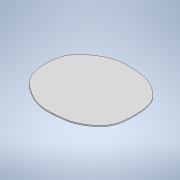
# Autodesk Inventor part: head_1
Saved by Autodesk Inventor 2020 (Build 240168000, 168)
## iProperties
Created: 2022-02-10
Part Number: head_1
Material: Типовые
Document SubType Name: Modeling
Designer: HP
Density: 1 g/cm^3
Appearance: По умолчанию
Author: HP
Autodesk Inventor part; units mm, degrees
ref_plane "YZ Plane" through (0, 0, 0) normal (1, 0, 0) x (0, 1, 0)
ref_plane "XZ Plane" through (0, 0, 0) normal (0, 1, 0) x (-1, 0, 0)
ref_plane "XY Plane" through (0, 0, 0) normal (0, 0, 1) x (1, 0, 0)
sketch "Эскиз1" plane through (0, 0, 0) normal (0, 1, 0) x (-1, 0, 0)
  line L0 (-81.3316, -22.101) -> (-82.4097, -10.5497) construction
  line L1 (-82.4097, -10.5497) -> (-83.3338, 3.774) construction
  line L2 (-83.3338, 3.774) -> (-82.2557, 21.486) construction
  line L3 (-82.2557, 21.486) -> (-81.3316, 38.8901) construction
  line L4 (-81.3316, 38.8901) -> (-79.8522, 51.3377) construction
  line L5 (-79.8522, 51.3377) -> (-76.1961, 64.7434) construction
  line L6 (-76.1961, 64.7434) -> (-73.0275, 74.6555) construction
  line L7 (-73.0275, 74.6555) -> (-68.2339, 84.2426) construction
  line L8 (-68.2339, 84.2426) -> (-63.1966, 91.2298) construction
  line L9 (-63.1966, 91.2298) -> (-56.2094, 98.7045) construction
  line L10 (-56.2094, 98.7045) -> (-49.8722, 104.8792) construction
  line L11 (-49.8722, 104.8792) -> (-42.6413, 111.5415) construction
  line L12 (-42.6413, 111.5415) -> (-35.4916, 118.0412) construction
  spline S0 degree 4 poles (-81.3316, -22.101) (-82.4097, -10.5497) (-83.3338, 3.774) (-82.2557, 21.486) (-81.3316, 38.8901) (-79.8522, 51.3377) (-76.1961, 64.7434) (-73.0275, 74.6555) (-68.2339, 84.2426) (-63.1966, 91.2298) (-56.2094, 98.7045) (-49.8722, 104.8792) (-42.6413, 111.5415) (-35.4916, 118.0412) knots 1 1 1 1 1 2 3 4 5 6 7 8 9 10 11 11 11 11 11
  line L13 (-35.4916, 118.0412) -> (-26.9213, 124.335) construction
  line L14 (-26.9213, 124.335) -> (-18.4284, 129.3436) construction
  line L15 (-18.4284, 129.3436) -> (-8.1934, 134.4974) construction
  line L16 (-8.1934, 134.4974) -> (-0.1361, 138.4897) construction
  line L17 (-0.1361, 138.4897) -> (9.5182, 142.1192) construction
  line L18 (9.5182, 142.1192) -> (19.245, 145.0227) construction
  line L19 (19.245, 145.0227) -> (26.7942, 146.4745) construction
  line L20 (26.7942, 146.4745) -> (34.6338, 147.7085) construction
  line L21 (34.6338, 147.7085) -> (42.183, 148.6521) construction
  line L22 (42.183, 148.6521) -> (49.8774, 149.6684) construction
  line L23 (49.8774, 149.6684) -> (59.0962, 150.9024) construction
  line L24 (59.0962, 150.9024) -> (68.823, 151.6283) construction
  line L25 (68.823, 151.6283) -> (77.4611, 152.2815) construction
  line L26 (77.4611, 152.2815) -> (85.0103, 152.2815) construction
  line L27 (85.0103, 152.2815) -> (93.1402, 152.9348) construction
  line L28 (93.1402, 152.9348) -> (101.4153, 152.9348) construction
  line L29 (101.4153, 152.9348) -> (111.5051, 151.5557) construction
  spline S1 degree 4 poles (-35.4916, 118.0412) (-26.9213, 124.335) (-18.4284, 129.3436) (-8.1934, 134.4974) (-0.1361, 138.4897) (9.5182, 142.1192) (19.245, 145.0227) (26.7942, 146.4745) (34.6338, 147.7085) (42.183, 148.6521) (49.8774, 149.6684) (59.0962, 150.9024) (68.823, 151.6283) (77.4611, 152.2815) (85.0103, 152.2815) (93.1402, 152.9348) (101.4153, 152.9348) (111.5051, 151.5557) knots 1 1 1 1 1 2 3 4 5 6 7 8 9 10 11 12 13 14 15 15 15 15 15
  line L30 (111.5051, 151.5557) -> (120.4722, 150.4408) construction
  line L31 (120.4722, 150.4408) -> (127.0223, 148.8843) construction
  line L32 (127.0223, 148.8843) -> (136.88, 145.7713) construction
  line L33 (136.88, 145.7713) -> (146.6728, 142.5287) construction
  line L34 (146.6728, 142.5287) -> (156.9196, 138.2484) construction
  line L35 (156.9196, 138.2484) -> (167.6204, 132.6061) construction
  line L36 (167.6204, 132.6061) -> (176.8944, 127.1585) construction
  line L37 (176.8944, 127.1585) -> (185.5199, 121.4514) construction
  line L38 (185.5199, 121.4514) -> (194.1438, 115.6177) construction
  spline S2 degree 4 poles (111.5051, 151.5557) (120.4722, 150.4408) (127.0223, 148.8843) (136.88, 145.7713) (146.6728, 142.5287) (156.9196, 138.2484) (167.6204, 132.6061) (176.8944, 127.1585) (185.5199, 121.4514) (194.1438, 115.6177) knots 1 1 1 1 1 2 3 4 5 6 7 7 7 7 7
  line L39 (194.1438, 115.6177) -> (200.24, 111.078) construction
  line L40 (200.24, 111.078) -> (206.9199, 106.0194) construction
  line L41 (206.9199, 106.0194) -> (214.1834, 99.9232) construction
  line L42 (214.1834, 99.9232) -> (219.8905, 93.2434) construction
  line L43 (219.8905, 93.2434) -> (226.1164, 84.3585) construction
  line L44 (226.1164, 84.3585) -> (232.2126, 74.7602) construction
  line L45 (232.2126, 74.7602) -> (234.0285, 71.4527) construction
  line L46 (234.0285, 71.4527) -> (236.5578, 65.162) construction
  line L47 (236.5578, 65.162) -> (240.1895, 53.5532) construction
  line L48 (240.1895, 53.5532) -> (243.1079, 38.7667) construction
  line L49 (243.1079, 38.7667) -> (244.9887, 26.8338) construction
  line L50 (244.9887, 26.8338) -> (246.2209, 14.4468) construction
  line L51 (246.2209, 14.4468) -> (246.2209, 2.9029) construction
  line L52 (246.2209, 2.9029) -> (245.2481, -13.7643) construction
  line L53 (245.2481, -13.7643) -> (243.7565, -27.3835) construction
  spline S3 degree 4 poles (194.1438, 115.6177) (200.24, 111.078) (206.9199, 106.0194) (214.1834, 99.9232) (219.8905, 93.2434) (226.1164, 84.3585) (232.2126, 74.7602) (234.0285, 71.4527) (236.5578, 65.162) (240.1895, 53.5532) (243.1079, 38.7667) (244.9887, 26.8338) (246.2209, 14.4468) (246.2209, 2.9029) (245.2481, -13.7643) (243.7565, -27.3835) knots 1 1 1 1 1 2 3 4 5 6 7 8 9 10 11 12 13 13 13 13 13
  line L54 (-83.3338, 3.774) -> (246.0649, 9.0912)
  line L55 (-82.1678, 29.7001) -> (-82.8725, 18.12) construction
  line L56 (-82.8725, 18.12) -> (-83.3338, 3.774) construction
  line L57 (-83.3338, 3.774) -> (-81.6846, -13.8941) construction
  line L58 (-81.6846, -13.8941) -> (-80.1992, -31.2592) construction
  line L59 (-80.1992, -31.2592) -> (-78.3188, -43.6526) construction
  line L60 (-78.3188, -43.6526) -> (-74.232, -56.9333) construction
  line L61 (-74.232, -56.9333) -> (-70.7451, -66.738) construction
  line L62 (-70.7451, -66.738) -> (-65.6446, -76.1654) construction
  line L63 (-65.6446, -76.1654) -> (-60.3844, -82.9864) construction
  line L64 (-60.3844, -82.9864) -> (-53.1596, -90.2316) construction
  line L65 (-53.1596, -90.2316) -> (-46.6263, -96.1986) construction
  line L66 (-46.6263, -96.1986) -> (-39.1841, -102.624) construction
  line L67 (-39.1841, -102.624) -> (-31.8284, -108.8896) construction
  spline S4 degree 4 poles (-82.1678, 29.7001) (-82.8725, 18.12) (-83.3338, 3.774) (-81.6846, -13.8941) (-80.1992, -31.2592) (-78.3188, -43.6526) (-74.232, -56.9333) (-70.7451, -66.738) (-65.6446, -76.1654) (-60.3844, -82.9864) (-53.1596, -90.2316) (-46.6263, -96.1986) (-39.1841, -102.624) (-31.8284, -108.8896) knots 1 1 1 1 1 2 3 4 5 6 7 8 9 10 11 11 11 11 11
  line L68 (-31.8284, -108.8896) -> (-23.0594, -114.9034) construction
  line L69 (-23.0594, -114.9034) -> (-14.4093, -119.6353) construction
  line L70 (-14.4093, -119.6353) -> (-4.0133, -124.4561) construction
  line L71 (-4.0133, -124.4561) -> (4.1687, -128.1863) construction
  line L72 (4.1687, -128.1863) -> (13.9351, -131.5022) construction
  line L73 (13.9351, -131.5022) -> (23.7506, -134.0903) construction
  line L74 (23.7506, -134.0903) -> (31.3427, -135.2977) construction
  line L75 (31.3427, -135.2977) -> (39.218, -136.278) construction
  line L76 (39.218, -136.278) -> (46.7937, -136.9775) construction
  line L77 (46.7937, -136.9775) -> (54.5169, -137.7449) construction
  line L78 (54.5169, -137.7449) -> (63.7707, -138.6807) construction
  line L79 (63.7707, -138.6807) -> (73.5159, -139.0922) construction
  line L80 (73.5159, -139.0922) -> (82.1705, -139.4664) construction
  line L81 (82.1705, -139.4664) -> (89.7158, -139.2227) construction
  line L82 (89.7158, -139.2227) -> (97.8626, -139.6133) construction
  line L83 (97.8626, -139.6133) -> (106.1334, -139.3462) construction
  line L84 (106.1334, -139.3462) -> (116.1734, -137.6421) construction
  spline S5 degree 4 poles (-31.8284, -108.8896) (-23.0594, -114.9034) (-14.4093, -119.6353) (-4.0133, -124.4561) (4.1687, -128.1863) (13.9351, -131.5022) (23.7506, -134.0903) (31.3427, -135.2977) (39.218, -136.278) (46.7937, -136.9775) (54.5169, -137.7449) (63.7707, -138.6807) (73.5159, -139.0922) (82.1705, -139.4664) (89.7158, -139.2227) (97.8626, -139.6133) (106.1334, -139.3462) (116.1734, -137.6421) knots 1 1 1 1 1 2 3 4 5 6 7 8 9 10 11 12 13 14 15 15 15 15 15
  line L85 (116.1734, -137.6421) -> (125.0998, -136.2383) construction
  line L86 (125.0998, -136.2383) -> (131.5963, -134.4712) construction
  line L87 (131.5963, -134.4712) -> (141.3484, -131.0417) construction
  line L88 (141.3484, -131.0417) -> (151.0315, -127.4847) construction
  line L89 (151.0315, -127.4847) -> (161.1348, -122.8759) construction
  line L90 (161.1348, -122.8759) -> (171.6479, -116.8912) construction
  line L91 (171.6479, -116.8912) -> (180.7412, -111.1471) construction
  line L92 (180.7412, -111.1471) -> (189.178, -105.1646) construction
  line L93 (189.178, -105.1646) -> (197.6091, -99.0555) construction
  spline S6 degree 4 poles (116.1734, -137.6421) (125.0998, -136.2383) (131.5963, -134.4712) (141.3484, -131.0417) (151.0315, -127.4847) (161.1348, -122.8759) (171.6479, -116.8912) (180.7412, -111.1471) (189.178, -105.1646) (197.6091, -99.0555) knots 1 1 1 1 1 2 3 4 5 6 7 7 7 7 7
  line L94 (197.6091, -99.0555) -> (203.5556, -94.3214) construction
  line L95 (203.5556, -94.3214) -> (210.0688, -89.0499) construction
  line L96 (210.0688, -89.0499) -> (217.1318, -82.7225) construction
  line L97 (217.1318, -82.7225) -> (222.6203, -75.8619) construction
  line L98 (222.6203, -75.8619) -> (228.5561, -66.7807) construction
  line L99 (228.5561, -66.7807) -> (234.3394, -56.9906) construction
  line L100 (234.3394, -56.9906) -> (236.0476, -53.6262) construction
  line L101 (236.0476, -53.6262) -> (238.3725, -47.2571) construction
  line L102 (238.3725, -47.2571) -> (241.6277, -35.5373) construction
  line L103 (241.6277, -35.5373) -> (244.0673, -20.6643) construction
  line L104 (244.0673, -20.6643) -> (245.5619, -8.6768) construction
  line L105 (245.5619, -8.6768) -> (246.3937, 3.7435) construction
  line L106 (246.3937, 3.7435) -> (246.0211, 15.2813) construction
  line L107 (246.0211, 15.2813) -> (244.5108, 31.9085) construction
  line L108 (244.5108, 31.9085) -> (242.5804, 45.4724) construction
  spline S7 degree 4 poles (197.6091, -99.0555) (203.5556, -94.3214) (210.0688, -89.0499) (217.1318, -82.7225) (222.6203, -75.8619) (228.5561, -66.7807) (234.3394, -56.9906) (236.0476, -53.6262) (238.3725, -47.2571) (241.6277, -35.5373) (244.0673, -20.6643) (245.5619, -8.6768) (246.3937, 3.7435) (246.0211, 15.2813) (244.5108, 31.9085) (242.5804, 45.4724) knots 1 1 1 1 1 2 3 4 5 6 7 8 9 10 11 12 13 13 13 13 13
  point P0 (0, 0)
  point P1 (245.5153, -7.5556)
  point P2 (246.0649, 9.0912)
  point P3 (244.9783, 25.7116)
  point P4 (-82.8445, 3.7819)
  constraints: 51 symmetric about line, 2 end point, 2 horizontal, 1 coincident, 1 vertical, 25 other
extrude "Выдавливание1" add sketch "Эскиз1" along normal blind 4 contours S0 S1 S2 S3 S7 L54 | L54 S3 S7 S6 S5 S4
